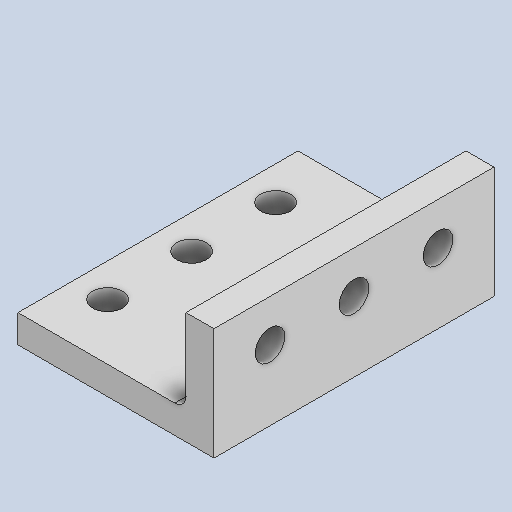
# Autodesk Inventor part: Linear Rail Frame Bracket
Saved by Autodesk Inventor 2022 (Build 260153000, 153)
## iProperties
Created: 2021-11-30
Part Number: Linear Rail Frame Bracket
Material: Generic
Document SubType Name: Modeling
Designer: efred
Density: 1 g/cm^3
Appearance: Default
Author: efred
Autodesk Inventor part; units mm, degrees
ref_plane "YZ Plane" through (0, 0, 0) normal (1, 0, 0) x (0, 1, 0)
ref_plane "XZ Plane" through (0, 0, 0) normal (0, 1, 0) x (-1, 0, 0)
ref_plane "XY Plane" through (0, 0, 0) normal (0, 0, 1) x (1, 0, 0)
sketch "Sketch1" plane through (0, 0, 0) normal (0, 0, 1) x (1, 0, 0)
  line L0 (25, 5.55) -> (-25, 5.55) construction
  line L1 (-25, 5.55) -> (-25, -5.55) construction
  line L2 (-25, -5.55) -> (25, -5.55) construction
  line L3 (25, -5.55) -> (25, 5.55) construction
  line L4 (25.1, -5.55) -> (25.1, 149.35) construction
  line L5 (25.1, -5.55) -> (35.1, -5.55) construction
  line L6 (35.1, -5.55) -> (35.1, 149.35) construction
  line L7 (25.1, 149.35) -> (35.1, 149.35) construction
  line L8 (25, 25.65) -> (25, 5.65)
  line L9 (25, 5.65) -> (-10, 5.65)
  line L10 (20, 25.65) -> (20, 10.65)
  line L11 (20, 10.65) -> (-10, 10.65)
  line L12 (20, 25.65) -> (25, 25.65)
  line L13 (-10, 10.65) -> (-10, 5.65)
  point P0 (0, 0)
  dimension "d0" = 0.1
  dimension "d1" = 0.1
  dimension "d2" = 5
  dimension "d3" = 35
  dimension "d4" = 20
  constraints: 12 end point, 2 horizontal, 1 horizontal alignment, 1 perpendicular, 1 vertical, 1 vertical alignment, 1 other
  measures "d0" distance between parallel lines of L4 L8
  measures "d1" distance between parallel lines of L0 L9
  measures "d2" distance between parallel lines of L9 L11
  measures "d3" distance of L8.end L9.end
  measures "d4" distance of L8.start L8.end
extrude "Extrusion1" add sketch "Sketch1" against normal blind 50
sketch "Sketch2" plane through (20, 10.65, 0) normal (-1, 0, 0) x (0, 0, 1)
  circle A0 centre (-40, 7.5) radius 2.65
  line L0 (-50, 0) -> (-50, 15) projected
  line L1 (-50, 7.5) -> (-0.7445, 7.5) construction
  line L2 (0, 15) -> (-50, 15) projected
  line L3 (-25, 15) -> (-25, 0) construction
  line L4 (0, 0) -> (-50, 0) projected
  circle A1 centre (-10, 7.5) radius 2.65
  circle A2 centre (-25, 7.5) radius 2.65
  point P0 (0, -10.65)
  dimension "d7" = 5.3
  dimension "d8" = 10
  dimension "d9" = 5.3
  constraints: 4 end point, 4 midpoint, 3 centre point, 1 horizontal, 1 point on line, 1 symmetric about line, 1 other
  measures "d7" diameter of A0
  measures "d8" distance from line of L0 A0.centre
  measures "d9" diameter of A2
extrude "Extrusion2" cut sketch "Sketch2" against normal through all
sketch "Sketch3" plane through (-10, 10.65, 0) normal (0, 1, 0) x (1, 0, 0)
  circle A0 centre (6, 10) radius 2.65
  line L0 (30, 0) -> (0, 0) projected
  line L1 (0, 0) -> (0, 50) projected
  line L2 (6, 0) -> (6, 49.4853) construction
  line L3 (0, 0) -> (0, 50) projected
  line L4 (0, 25) -> (30, 25) construction
  line L5 (30, 22.35) -> (30, 27.65) projected
  circle A1 centre (6, 40) radius 2.65
  circle A2 centre (6, 25) radius 2.65
  point P0 (10, 0)
  dimension "d12" = 5.3
  dimension "d13" = 10
  dimension "d14" = 6
  dimension "d15" = 5.3
  constraints: 4 end point, 4 point on line, 3 centre point, 2 midpoint, 1 symmetric about line, 1 vertical, 1 other
  measures "d12" diameter of A0
  measures "d13" distance from line of L0 A0.centre
  measures "d14" distance from line of L1 A0.centre
  measures "d15" diameter of A2
extrude "Extrusion3" cut sketch "Sketch3" against normal through all
fillet "Fillet1" radius 2 1 edges at (20, 10.65, -25)
equation "\"d9\" = d7"
equation "\"d15\" = d12"
body "Solid1"
